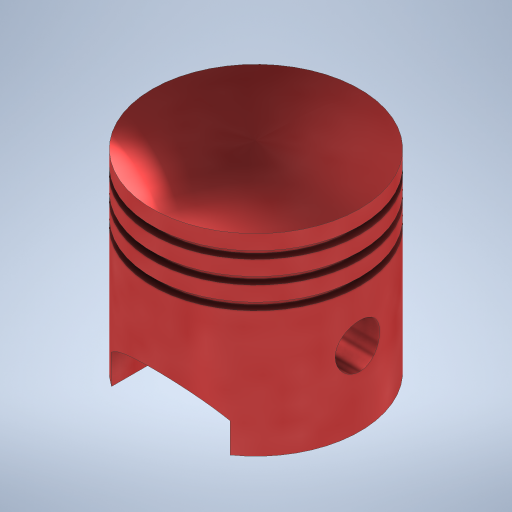
# Autodesk Inventor part: Piston
Saved by Autodesk Inventor 2023 (Build 270158000, 158)
## iProperties
Created: 2023-10-06
Part Number: Piston
Material: Generic
Document SubType Name: Modeling
Designer: huy20
Density: 1 g/cm^3
Appearance: Steel - Polished
Author: huy20
Autodesk Inventor part; units mm, degrees
ref_plane "XZ Plane" through (0, 0, 0) normal (0, 1, 0) x (-1, 0, 0)
ref_plane "XY Plane" through (0, 0, 0) normal (0, 0, 1) x (1, 0, 0)
sketch "Sketch1" plane through (0, 0, 0) normal (0, 0, 1) x (1, 0, 0)
  line L0 (0, 0) -> (0, 17.8408)
  line L1 (6.9963, 13) -> (0, 13) construction
  arc A0 (6.9963, 13) -> (0, 13.5) centre (-1.878, -61.9766) ccw
  line L2 (4.9963, 0) -> (4.9963, 12)
  line L3 (4.9963, 12) -> (0, 12)
  line L4 (6.9963, 12) -> (6.5, 12)
  line L5 (6.5, 12) -> (6.5, 11.5)
  line L6 (6.5, 11.5) -> (7, 11.5)
  line L7 (7, 10.5) -> (6.5, 10.5)
  line L8 (6.5, 10.5) -> (6.5, 10)
  line L9 (6.5, 10) -> (7, 10)
  line L10 (7, 9) -> (6.5, 9)
  line L11 (6.5, 9) -> (6.5, 8.5)
  line L12 (6.5, 8.5) -> (7, 8.5)
  line L13 (6.9963, 12) -> (6.9963, 13)
  line L14 (7, 10.5) -> (7, 11.5)
  line L15 (7, 0) -> (7, 8.5)
  line L16 (7, 9) -> (7, 10)
  line L17 (4.9963, 0) -> (7, 0)
  point P0 (6.5, 11.75)
  point P1 (6.7482, 12)
  point P2 (6.5, 10.25)
  point P3 (6.75, 10.5)
  point P4 (6.5, 8.75)
  point P5 (6.75, 9)
  dimension "d0" = 13
  dimension "d2" = 0.5
  dimension "d4" = 1
  dimension "d6" = 0.5
  dimension "d7" = 0.5
  dimension "d8" = 0.5
  dimension "d9" = 1
  dimension "d10" = 1
  dimension "d29" = 75.5
  dimension "d30" = 14
  constraints: 36 end point, 9 perpendicular, 6 midpoint, 6 vertical, 4 horizontal, 3 point on line, 2 point on circle, 1 centre point
  measures "d0" distance of L15.start L1.start
  measures "d2" distance of L1.end A0.end
  measures "d4" distance between parallel lines of L3 L1
  measures "d6" distance from line of L6 point (6.748, 12)
  measures "d7" distance from line of L9 point (6.75, 10.5)
  measures "d8" distance from line of L12 point (6.75, 9)
  measures "d9" distance between parallel lines of L7 L6
  measures "d10" distance between parallel lines of L10 L9
  measures "d29" radius of A0
  measures "d30" diameter of L15 L0
revolve "Revolution1" add sketch "Sketch1" angle 360 about axis through (0, 0, 0) along (0, 1, 0)
sketch "Sketch2" plane through (0, 0, 0) normal (0, 0, 1) x (1, 0, 0)
  line L0 (-4, 0) -> (-4, 2)
  line L1 (4, 2) -> (4, 0)
  line L2 (-4, 0) -> (4, 0)
  line L3 (4.9963, 0) -> (-4.9963, 0) construction
  arc A0 (4, 2) -> (-4, 2) centre (0, -1.8677) ccw
  point P0 (0, 0)
  point P1 (0, 0)
  point P2 (0, 0)
  dimension "d12" = 4
  dimension "d13" = 4
  dimension "d14" = 2
  constraints: 6 end point, 2 midpoint, 2 point on circle, 2 vertical, 1 centre point, 1 coincident, 1 horizontal, 1 parallel
  measures "d12" distance from line of point (0, 0) L1
  measures "d13" distance from line of L0 point (0, 0)
  measures "d14" distance of L1.start L1.end
extrude "Extrusion1" cut sketch "Sketch2" along normal through all both and the other way through all
sketch "Sketch3" plane through (0, 0, 0) normal (1, 0, 0) x (0, 1, 0)
  circle A0 centre (5, 0) radius 1.5
  point P0 (0, 0)
  dimension "d17" = 5
  dimension "d18" = 3
  constraints: 1 centre point
  measures "d17" distance of point (0, 0) A0.centre
  measures "d18" diameter of A0
extrude "Extrusion2" cut sketch "Sketch3" along normal through all both and the other way through all
ref_plane "Work Plane1" through (3, 0, 0) normal (1, 0, 0) x (0, 1, 0)
sketch "Sketch4" plane through (3, 0, 0) normal (1, 0, 0) x (0, 1, 0)
  circle A0 centre (5, 0) radius 1.5
  circle A1 centre (5, 0) radius 2
  point P0 (0, 0)
  dimension "d22" = 4
  dimension "d23" = 5
  dimension "d24" = 3
  dimension "d25" = 1.5
  constraints: 2 centre point, 1 coincident, 1 other
  measures "d22" diameter of A1
  measures "d23" distance of point (0, 0) A0.centre
  measures "d24" diameter of A0
  measures "d25" distance of point (5, -1.5) A0.centre
extrude "Extrusion3" add sketch "Sketch4" along normal up to surface round surface about axis through (0, 6, 0) along (0, 1, 0) radius 4.9963 far side no
mirror "Mirror1" about plane through (0, 0, 0) normal (1, 0, 0) of "Extrusion3"
body "Solid1"
